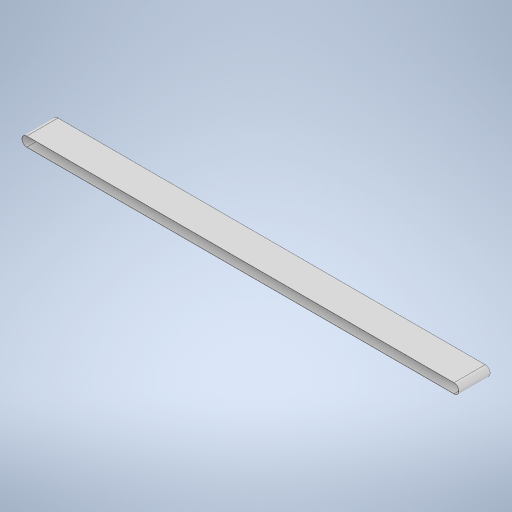
# Autodesk Inventor part: BandaLona
Saved by Autodesk Inventor 2024 (Build 280153000, 153)
## iProperties
Created: 2024-06-28
Part Number: BandaLona
Material: Genérico
Document SubType Name: Modeling
Designer: USER
Density: 1 g/cm^3
Appearance: Valor por defecto
Author: USER
Autodesk Inventor part; units mm, degrees
ref_plane "YZ Plane" through (0, 0, 0) normal (1, 0, 0) x (0, 1, 0)
ref_plane "XZ Plane" through (0, 0, 0) normal (0, 1, 0) x (-1, 0, 0)
ref_plane "XY Plane" through (0, 0, 0) normal (0, 0, 1) x (1, 0, 0)
sketch "Boceto1" plane through (0, 0, 0) normal (0, 0, 1) x (1, 0, 0)
  line L0 (-2850, 250.9244) -> (10850, 250.9244)
  line L1 (10850, 250.9244) -> (10850, -49.0756) construction
  line L2 (10850, -49.0756) -> (-2850, -49.0756)
  line L3 (-2850, -49.0756) -> (-2850, 250.9244) construction
  line L4 (-2850, 250.9244) -> (10850, -49.0756) construction
  line L5 (10850, 250.9244) -> (-2850, -49.0756) construction
  arc A0 (10850, -49.0756) -> (10850, 250.9244) centre (10850, 100.9244) ccw
  arc A1 (-2850, 250.9244) -> (-2850, -49.0756) centre (-2850, 100.9244) ccw
  arc A2 (10850, -56.0756) -> (10850, 257.9244) centre (10850, 100.9244) ccw
  line L6 (10850, -56.0756) -> (-2850, -56.0756)
  arc A3 (-2850, 257.9244) -> (-2850, -56.0756) centre (-2850, 100.9244) ccw
  line L7 (-2850, 257.9244) -> (10850, 257.9244)
  point P0 (-650, 3378.1666)
  point P1 (4000, 100.9244)
  dimension "d11" = 13700
  dimension "d12" = 7
  dimension "d13" = 300
  constraints: 16 end point, 8 point on circle, 4 centre point, 4 midpoint, 3 parallel, 1 horizontal, 1 perpendicular, 3 other
  measures "d11" distance of L2.end L1.end
  measures "d12" distance between parallel lines of L0 L7
  measures "d13" distance between parallel lines of L2 L0
extrude "Extrusión1" add sketch "Boceto1" along normal blind 1000
equation "\"L\" = 14000"
